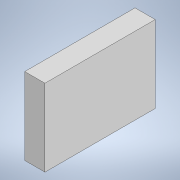
# Autodesk Inventor part: Part2113
Saved by Autodesk Inventor 2022 (Build 260153070, 153G)
## iProperties
Created: 2021-07-09
Part Number: Part2113
Material: Generic
Document SubType Name: Modeling
Designer: sachin
Density: 1 g/cm^3
Appearance: Default
Author: sachin
Autodesk Inventor part; units mm, degrees
ref_plane "YZ Plane" through (0, 0, 0) normal (1, 0, 0) x (0, 1, 0)
ref_plane "XZ Plane" through (0, 0, 0) normal (0, 1, 0) x (-1, 0, 0)
ref_plane "XY Plane" through (0, 0, 0) normal (0, 0, 1) x (1, 0, 0)
sketch "Sketch1" plane through (0, 0, 0) normal (1, 0, 0) x (0, 1, 0)
  line L0 (81.4953, 141.6803) -> (28.2844, 141.6803)
  line L1 (28.2844, 141.6803) -> (28.2844, 65.4803)
  line L2 (28.2844, 65.4803) -> (81.4953, 65.4803)
  line L3 (81.4953, 65.4803) -> (81.4953, 141.6803)
  point P0 (0, 0)
  dimension "d0" = 76.2
  dimension "d1" = 53.2109
  constraints: 8 end point, 2 parallel, 1 horizontal, 1 perpendicular
  measures "d0" distance of L2.end L0.start
  measures "d1" distance of L1.end L2.end
extrude "Extrusion1" add sketch "Sketch1" along normal blind 13.97
body "Solid1"
